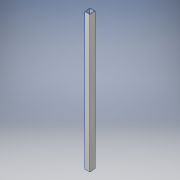
# Autodesk Inventor part: Turret Support Extrusion
Saved by Autodesk Inventor 2019.4 (Build 234330000, 330)
## iProperties
Created: 2020-01-11
Part Number: Turret Support Extrusion
Material: Aluminum 6061
Document SubType Name: Modeling
Designer: admin
Density: 2.7 g/cm^3
Appearance: Aluminum - Flat
Author: admin
Autodesk Inventor part; units mm, degrees
ref_plane "YZ Plane" through (0, 0, 0) normal (1, 0, 0) x (0, 1, 0)
ref_plane "XZ Plane" through (0, 0, 0) normal (0, 1, 0) x (-1, 0, 0)
ref_plane "XY Plane" through (0, 0, 0) normal (0, 0, 1) x (1, 0, 0)
sketch "Sketch1" plane through (0, 0, 0) normal (0, 1, 0) x (-1, 0, 0)
  line L0 (-10, 10) -> (10, 10)
  line L1 (10, 10) -> (10, -10)
  line L2 (10, -10) -> (-10, -10)
  line L3 (-10, -10) -> (-10, 10)
  line L4 (-10, 10) -> (10, -10) construction
  line L5 (10, 10) -> (-10, -10) construction
  line L6 (8, -8) -> (8, 8)
  line L7 (8, 8) -> (-8, 8)
  line L8 (-8, 8) -> (-8, -8)
  line L9 (-8, -8) -> (8, -8)
  point P0 (0, 0)
  dimension "d0" = 20
  dimension "d1" = 20
  dimension "d2" = 2
  constraints: 20 end point, 4 parallel, 2 midpoint, 2 perpendicular, 1 horizontal, 3 other
  measures "d0" distance of L1.end L2.end
  measures "d1" distance of L0.end L1.end
  measures "d2" distance between parallel lines of L1 L6
extrude "Extrusion1" add sketch "Sketch1" along normal blind 550
sketch "Sketch2" plane through (10, 0, 10) normal (1, 0, 0) x (0, 0, -1)
  line L0 (0, 0) -> (0, 550) projected
  line L1 (0, 0) -> (20, 2.261)
  line L2 (20, 0) -> (20, 550) projected
  line L3 (0, 523.3124) -> (20, 525.5735)
  line L4 (20, 525.5735) -> (78.4148, 8.8649) construction
  line L5 (78.4148, 8.8649) -> (20, 2.261) construction
  line L6 (0, 550) -> (20, 550) projected
  line L7 (20, 0) -> (0, 0) projected
  point P0 (10, 0)
  dimension "d5" = 83.55
  dimension "d6" = 83.55
  dimension "d7" = 520
  constraints: 8 end point, 3 point on line, 1 collinear, 1 perpendicular
  measures "d5" angle of L0 L1
  measures "d6" angle of L0 L3
  measures "d7" distance of L3.end L4.end
extrude "Extrusion2" cut sketch "Sketch2" against normal through all contours L1 L2 L7 | L0 L6 L2 L3
body "Solid1"
